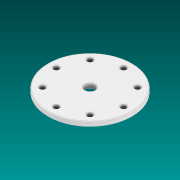
# Autodesk Inventor part: endeffector mount as 8 compact
Saved by Autodesk Inventor 2020.3 (Build 243373000, 373)
## iProperties
Created: 2020-05-18
Part Number: endeffector mount as 8 compact
Material: ABS Plastic
Document SubType Name: Modeling
Designer: stefa
Density: 1.06 g/cm^3
Appearance: Smooth - White
Mass: 15.5843 g
Surface Area: 85.8038 cm^2
Volume: 14.7021 cm^3
Author: stefa
Autodesk Inventor part; units mm, degrees
ref_plane "YZ Plane" through (0, 0, 0) normal (1, 0, 0) x (0, 1, 0)
ref_plane "XZ Plane" through (0, 0, 0) normal (0, 1, 0) x (-1, 0, 0)
sketch "Sketch1" plane through (0, 0, 0) normal (0, 1, 0) x (-1, 0, 0)
  circle A0 centre (0, 0) radius 4
  circle A1 centre (0, 0) radius 35
  circle A2 centre (0, -28) radius 2
  circle A3 centre (19.799, -19.799) radius 2
  circle A4 centre (28, 0) radius 2
  circle A5 centre (19.799, 19.799) radius 2
  circle A6 centre (0, 28) radius 2
  circle A7 centre (-19.799, 19.799) radius 2
  circle A8 centre (-28, 0) radius 2
  circle A9 centre (-19.799, -19.799) radius 2
  dimension "d0" = 70
  dimension "d1" = 8
  dimension "d4" = 4
  dimension "d5" = 28
  dimension "d8" = 360
  dimension "d21" = 21.4303
  constraints: 10 centre point, 2 coincident, 1 vertical alignment, 17 other
  measures "d0" diameter of A1
  measures "d1" diameter of A0
  measures "d4" diameter of A2
  measures "d5" distance of A2.centre point (0, 0)
  measures "d21" distance of A3.centre A4.centre
extrude "Extrusion1" add sketch "Sketch1" along normal blind 4
ref_plane "Work Plane2" through (0, 0, 0) normal (0.3826834, 0, 0.9238795) x (0, 1, 0)
thread "Thread2" size "M4x0.7" class "6H" standard "ANSI Metric M Profile" full length
thread "Thread3" size "M4x0.7" class "6H" standard "ANSI Metric M Profile" full length
thread "Thread4" size "M4x0.7" class "6H" standard "ANSI Metric M Profile" full length
thread "Thread5" size "M4x0.7" class "6H" standard "ANSI Metric M Profile" full length
thread "Thread6" size "M4x0.7" class "6H" standard "ANSI Metric M Profile" full length
thread "Thread7" size "M4x0.7" class "6H" standard "ANSI Metric M Profile" full length
thread "Thread8" size "M4x0.7" class "6H" standard "ANSI Metric M Profile" full length
thread "Thread9" size "M4x0.7" class "6H" standard "ANSI Metric M Profile" full length
chamfer "Chamfer2" distance 0.5 angle 45 20 edges at (30, 0, 0) (21.799, 4, 19.799) (30, 4, 0) (21.799, 0, 19.799) (35, 0, 0) (4, 0, 0) (4, 4, 0) (2, 0, 28) (2, 4, 28) (21.799, 0, -19.799) (21.799, 4, -19.799) (-17.799, 0, 19.799) (-17.799, 4, 19.799) (35, 4, 0) (-26, 0, 0) (-26, 4, 0) (2, 0, -28) (2, 4, -28) (-17.799, 0, -19.799) (-17.799, 4, -19.799)
body "Solid1"
